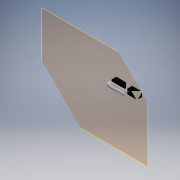
# Autodesk Inventor part: fuse
Saved by Autodesk Inventor 2016 (Build 200138000, 138)
## iProperties
Created: 2016-04-08
Part Number: fuse
Material: Generic
Document SubType Name: Modeling
Designer: Paschalis
Density: 1 g/cm^3
Appearance: Default
Author: Paschalis
Autodesk Inventor part; units mm, degrees
ref_plane "YZ Plane" through (0, 0, 0) normal (1, 0, 0) x (0, 1, 0)
ref_plane "XZ Plane" through (0, 0, 0) normal (0, 1, 0) x (-1, 0, 0)
ref_plane "XY Plane" through (0, 0, 0) normal (0, 0, 1) x (1, 0, 0)
ref_plane "Work Plane1" through (0, 0, 0) normal (0, 0, 1) x (1, 0, 0)
sketch "Sketch1" plane through (0, 0, 0) normal (0, 0, 1) x (1, 0, 0)
  circle A0 centre (23.98, 18.1) radius 0.8 projected
  circle A1 centre (47.16, 18.1) radius 0.8 projected
  circle A2 centre (40.4, 18.1) radius 0.8 projected
  circle A3 centre (30.74, 18.1) radius 0.8 projected
  line L0 (22.39, 20.64) -> (32.55, 20.64)
  line L1 (32.55, 20.64) -> (32.55, 15.56)
  line L2 (32.55, 15.56) -> (22.39, 15.56)
  line L3 (22.39, 15.56) -> (22.39, 20.64)
  circle A4 centre (27.47, 18.1025) radius 0.3 projected
  circle A5 centre (43.98, 16.8325) radius 0.3 projected
  line L4 (38.81, 20.64) -> (48.97, 20.64)
  line L5 (48.97, 20.64) -> (48.97, 15.56)
  line L6 (48.97, 15.56) -> (38.81, 15.56)
  line L7 (38.81, 15.56) -> (38.81, 20.64)
  point P0 (0, 0)
  point P1 (32.55, 18.1)
  point P2 (27.47, 20.64)
  dimension "d0" = 5.08
  dimension "d1" = 10.16
  dimension "d2" = 5.08
  dimension "d3" = 10.16
  constraints: 16 end point, 4 parallel, 2 horizontal, 2 midpoint, 2 perpendicular, 1 horizontal alignment, 1 vertical alignment
  measures "d0" distance of L0.end L1.end
  measures "d1" distance of L0.start L0.end
  measures "d2" distance of L4.end L6.start
  measures "d3" distance of L4.start L4.end
extrude "Extrusion1" add sketch "Sketch1" along normal blind 5 contours A0 | A1 | A2 | A3 | L0 L1 L2 L3 | A4 | A5 | L4 L5 L6 L7
sketch "Sketch2" plane through (48.97, 15.56, 0) normal (1, 0, 0) x (0, 0, -1)
  line L0 (0, 5.08) -> (0, 0) projected
  line L1 (0, 5.08) -> (-5, 5.08) projected
  line L2 (-5, 0) -> (-5, 5.08) projected
  line L3 (0, 0) -> (-5, 0) projected
  circle A0 centre (-7.5, 2.54) radius 2.5
  point P0 (0, -15.56)
  point P1 (-5, 2.54)
  dimension "d6" = 5
  dimension "d7" = 2.5
  constraints: 1 centre point, 1 horizontal alignment, 1 midpoint
  measures "d6" diameter of A0
  measures "d7" distance of point (-5, 2.54) A0.centre
extrude "Extrusion2" add sketch "Sketch2" against normal up to surface (26.58 mm away) contours A0
body "Solid1"
